syringe_puller_v1 (Autodesk Fusion 360 design; units mm, degrees)
Autodesk Fusion 360 part; units mm, degrees
sketch "Sketch1" plane through (0, 0, 0) normal (0, 0, 1) x (1, 0, 0)
  line L0 (16, 3.5) -> (-16, 3.5)
  line L1 (-16, 3.5) -> (-16, -3.5)
  line L2 (-16, -3.5) -> (16, -3.5)
  line L3 (16, -3.5) -> (16, 3.5)
  line L4 (16, 3.5) -> (-16, -3.5) construction
  line L5 (-16, 3.5) -> (16, -3.5) construction
  dimension "d1" = 7
  dimension "d2" = 32
  constraint horizontal L0
  constraint perpendicular L0 L1
  constraint parallel L0 L2
  constraint parallel L1 L3
  constraint coincident L4 origin
  constraint coincident L5 origin
  measures "d1" distance of L0.end L1.end
  measures "d2" distance of L0.start L0.end
extrude "Extrude1" add sketch "Sketch1" along normal blind 6
sketch "Sketch2" plane through (0, 3.5, 0) normal (0, 1, 0) x (-1, 0, 0)
  line L0 (-16, 0) -> (16, 0)
  line L1 (16, 0) -> (16, 6)
  line L2 (16, 6) -> (-16, 6)
  line L3 (-16, 6) -> (-16, 0)
  spline S0 degree 5 poles (-7.1322, 6) (-7.3673, 6) (-7.8114, 5.9542) (-8.3999, 5.7479) (-9.0471, 5.2296) (-9.7248, 4.3513) (-10.3869, 3.4588) (-11.1357, 2.7606) (-12.0283, 2.4083) (-13.0413, 2.4414) (-14.1039, 2.8325) (-14.9234, 3.3859) (-15.4861, 3.911) (-15.8334, 4.3063) (-16, 4.5153) knots 0 0 0 0 0 0 0.1 0.2 0.3 0.4 0.5 0.6 0.7 0.8 0.9 1 1 1 1 1 1
  line L4 (-6.288, 6) -> (-7.9764, 6)
  line L5 (-15.3842, 3.743) -> (-16.6158, 5.2877)
  point P0 (-11.1746, 2.8439)
  constraint coincident L2 S0.start
  constraint midpoint S0.start L4
  constraint collinear L2 L4
  constraint midpoint S0.end L5
  constraint coincident L3 S0.end
extrude "Extrude2" cut sketch "Sketch2" against normal through all contours L2 L3 S0 L4
fillet "Fillet1" radius 0.5 1 edges at (16, 0, 4.5153)
